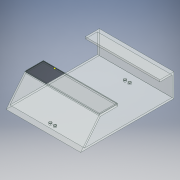
# Autodesk Inventor part: Bottom Plastic
Saved by Autodesk Inventor 2018 (Build 220112000, 112)
## iProperties
Created: 2018-02-19
Part Number: Bottom Plastic
Material: Generic
Document SubType Name: Modeling
Designer: Melda
Density: 1 g/cm^3
Appearance: Clear
Author: Melda
Autodesk Inventor part; units mm, degrees
ref_plane "YZ Plane" through (0, 0, 0) normal (1, 0, 0) x (0, 1, 0)
ref_plane "XZ Plane" through (0, 0, 0) normal (0, 1, 0) x (-1, 0, 0)
ref_plane "XY Plane" through (0, 0, 0) normal (0, 0, 1) x (1, 0, 0)
sketch "Sketch1" plane through (0, 0, 0) normal (1, 0, 0) x (0, 1, 0)
  point P0 (0, 0)
sketch "Sketch2" plane through (0, 0, 0) normal (1, 0, 0) x (0, 1, 0)
  line L0 (25.8289, -95.4545) -> (-24.1711, -95.4545)
  line L1 (-24.1711, -95.4545) -> (-24.1711, 104.5455)
  line L2 (-24.1711, 104.5455) -> (25.8289, 64.5455)
  line L3 (25.8289, 64.5455) -> (25.8289, 24.5455)
  line L4 (25.8289, -95.4545) -> (25.8289, -65.4545)
  line L5 (21.8289, -91.4545) -> (-20.1711, -91.4545)
  line L6 (-20.1711, -91.4545) -> (-20.1711, 24.5455)
  line L7 (21.8289, 62.623) -> (-20.1711, 96.223)
  line L8 (-20.1711, 96.223) -> (-20.1711, 24.5455)
  line L9 (25.8289, 24.5455) -> (21.8289, 24.5455)
  line L10 (25.8289, -65.4545) -> (21.8289, -65.4545)
  line L11 (21.8289, 62.623) -> (21.8289, 24.5455)
  line L12 (21.8289, -65.4545) -> (21.8289, -91.4545)
  point P0 (0, 0)
  dimension "d3" = 200
  dimension "d4" = 40
  dimension "d5" = 50
  dimension "d6" = 30
  dimension "d7" = 40
  dimension "d9" = 51.34
  dimension "d10" = 4
  dimension "d12" = 4
  dimension "d14" = 4
  dimension "d15" = 4
  dimension "d16" = 4
  dimension "d17" = 4
  dimension "d18" = 4
  constraints: 26 end point, 5 perpendicular, 4 parallel, 2 vertical, 1 horizontal, 1 point on line
  measures "d3" distance of L0.end L1.end
  measures "d4" vertical distance of L1.end L2.end
  measures "d5" distance of L0.start L0.end
  measures "d6" distance of L0.start L4.end
  measures "d7" distance of L2.end L3.end
  measures "d9" angle of L1 L2
  measures "d10" distance of L4.end L10.end
  measures "d12" distance between parallel lines of L1 L6
  measures "d14" distance from line of L2 L7.end
  measures "d15" distance of L3.end L9.end
  measures "d16" distance from line of L2 L7.start
  measures "d17" distance from line of L0 L5.start
  measures "d18" distance from line of L0 L5.end
extrude "Extrusion1" add sketch "Sketch2" along normal blind 160
sketch "Sketch3" plane through (0, 25.8289, 64.5455) normal (0, 1, 0) x (1, 0, 0)
  line L0 (1, 1) -> (159, 1)
  line L1 (159, 1) -> (159, 39)
  line L2 (159, 39) -> (1, 39)
  line L3 (1, 39) -> (1, 1)
  line L4 (0, 40) -> (0, 0) projected
  line L5 (0, 40) -> (160, 40) projected
  line L6 (0, 0) -> (160, 0) projected
  line L7 (160, 40) -> (160, 0) projected
  point P0 (0, 64.5455)
  dimension "d21" = 1
  dimension "d22" = 1
  dimension "d23" = 1
  dimension "d24" = 1
  constraints: 8 end point, 6 parallel, 1 horizontal, 1 perpendicular
  measures "d21" distance between parallel lines of L4 L3
  measures "d22" distance between parallel lines of L5 L2
  measures "d23" distance between parallel lines of L6 L0
  measures "d24" distance between parallel lines of L7 L1
extrude "Extrusion2" add sketch "Sketch3" along normal blind 2 contours L3 L2 L1 L0
sketch "Sketch5" plane through (0, 0, 0) normal (-1, 0, 0) x (0, 0, 1)
  point P0 (0, 0)
sketch "Sketch6" plane through (0, -24.1711, -95.4545) normal (0, -1, 0) x (1, 0, 0)
  circle A0 centre (75, 180) radius 2.5
  circle A1 centre (75, 180) radius 3
  line L0 (0, 200) -> (160, 200) projected
  line L1 (0, 200) -> (0, 0) projected
  circle A2 centre (85, 180) radius 2.5
  circle A3 centre (85, 180) radius 3
  circle A4 centre (85, 20) radius 2.5
  circle A5 centre (85, 20) radius 3
  circle A6 centre (75, 20) radius 2.5
  circle A7 centre (75, 20) radius 3
  line L2 (160, 200) -> (160, 0) projected
  line L3 (0, 0) -> (160, 0) projected
  point P0 (0, 95.4545)
  dimension "d33" = 5
  dimension "d34" = 6
  dimension "d35" = 20
  dimension "d36" = 75
  dimension "d37" = 5
  dimension "d38" = 6
  dimension "d39" = 5
  dimension "d40" = 6
  dimension "d41" = 5
  dimension "d42" = 6
  dimension "d43" = 75
  dimension "d44" = 20
  dimension "d45" = 20
  dimension "d46" = 20
  dimension "d47" = 75
  dimension "d48" = 75
  constraints: 8 centre point, 4 coincident
  measures "d33" diameter of A0
  measures "d34" diameter of A1
  measures "d35" distance from line of L0 A1.centre
  measures "d36" distance from line of L1 A1.centre
  measures "d37" diameter of A2
  measures "d38" diameter of A3
  measures "d39" diameter of A4
  measures "d40" diameter of A5
  measures "d41" diameter of A6
  measures "d42" diameter of A7
  measures "d43" distance from line of L2 A3.centre
  measures "d44" distance from line of L0 A3.centre
  measures "d45" distance from line of L3 A5.centre
  measures "d46" distance from line of L3 A7.centre
  measures "d47" distance from line of L2 A5.centre
  measures "d48" distance from line of L1 A7.centre
extrude "Extrusion4" cut sketch "Sketch6" against normal blind 3 contours A1 | A3 | A5 | A7
fillet "Fillet1" radius 2 4 edges at (72.5, -24.1711, -75.4545) (82.5, -24.1711, -75.4545) (72.5, -24.1711, 84.5455) (82.5, -24.1711, 84.5455)
body "Solid1"
